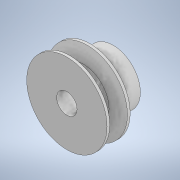
# Autodesk Inventor part: porra nenhuma
Saved by Autodesk Inventor 2022.1 (Build 261234020, 234B)
## iProperties
Created: 2023-07-21
Part Number: porra nenhuma
Material: Generic
Document SubType Name: Modeling
Designer: SENAI
Density: 1 g/cm^3
Appearance: Default
Author: SENAI
Autodesk Inventor part; units mm, degrees
ref_plane "YZ Plane" through (0, 0, 0) normal (1, 0, 0) x (0, 1, 0)
ref_plane "XZ Plane" through (0, 0, 0) normal (0, 1, 0) x (-1, 0, 0)
ref_plane "XY Plane" through (0, 0, 0) normal (0, 0, 1) x (1, 0, 0)
sketch "Sketch1" plane through (0, 0, 0) normal (0, 0, 1) x (1, 0, 0)
  circle A0 centre (17.8, 18.8069) radius 20
  circle A1 centre (17.8, 18.8069) radius 7.5
  point P0 (0, 0)
  dimension "d0" = 40
  dimension "d1" = 15
  constraints: 2 centre point, 1 coincident
  measures "d0" diameter of A0
  measures "d1" diameter of A1
extrude "Extrusion1" add sketch "Sketch1" along normal blind 17
sketch "Sketch2" plane through (17.8, 18.8069, 0) normal (0, 0, -1) x (-1, 0, 0)
  point P0 (17.8, -18.8069)
sketch "Sketch3" plane through (17.8, 18.8069, 17) normal (0, 0, 1) x (1, 0, 0)
  circle A0 centre (0, 0) radius 29.5
  point P0 (-17.8, -18.8069)
  dimension "d4" = 59
  constraints: 1 centre point
  measures "d4" diameter of A0
extrude "Extrusion2" add sketch "Sketch3" along normal blind 5
sketch "Sketch4" plane through (17.8, 18.8069, 17) normal (0, 0, -1) x (-1, 0, 0)
  circle A0 centre (0, 0) radius 8.6163
  point P0 (17.8, -18.8069)
  constraints: 1 centre point
sketch "Sketch5" plane through (17.8, 18.8069, 22) normal (0, 0, 1) x (1, 0, 0)
  circle A0 centre (0, 0) radius 7.5
  point P0 (-17.8, -18.8069)
  constraints: 1 centre point
extrude "Extrusion3" cut sketch "Sketch5" against normal blind 57.5
sketch "Sketch6" plane through (17.8, 18.8069, 17) normal (0, 0, -1) x (-1, 0, 0)
  point P0 (17.8, -18.8069)
sketch "Sketch7" plane through (17.8, 18.8069, 22) normal (0, 0, 1) x (1, 0, 0)
  point P0 (-17.8, -18.8069)
sketch "Sketch8" plane through (17.8, 18.8069, 22) normal (0, 0, 1) x (1, 0, 0)
  circle A0 centre (0, 0) radius 19
  point P0 (-17.8, -18.8069)
  dimension "d9" = 38
  constraints: 1 centre point
  measures "d9" diameter of A0
extrude "Extrusion4" add sketch "Sketch8" along normal blind 7
sketch "Sketch9" plane through (17.8, 18.8069, 29) normal (0, 0, 1) x (1, 0, 0)
  circle A0 centre (0, 0) radius 29.5
  point P0 (-17.8, -18.8069)
  constraints: 1 centre point
extrude "Extrusion5" add sketch "Sketch9" along normal blind 5
sketch "Sketch10" plane through (17.8, 18.8069, 22) normal (0, 0, -1) x (-1, 0, 0)
  circle A0 centre (0, 0) radius 7.5 projected
  circle A1 centre (0, 0) radius 7.5
  point P0 (17.8, -18.8069)
  constraints: 1 centre point, 1 coincident
sketch "Sketch11" plane through (17.8, 18.8069, 34) normal (0, 0, 1) x (1, 0, 0)
  circle A0 centre (0, 0) radius 7.5
  point P0 (-17.8, -18.8069)
  constraints: 1 centre point
extrude "Extrusion6" cut sketch "Sketch11" against normal blind 76.5
chamfer "Chamfer1" distance 3 distance2 10.5 1 edges at (-11.7, 18.8069, 29) measured on face at (47.2043, 16.4331, 32.3333)
chamfer "Chamfer2" distance 3 distance2 10.5 1 edges at (-11.7, 18.8069, 22) measured on face at (47.2043, 16.4331, 20.3333)
body "Solid1"
